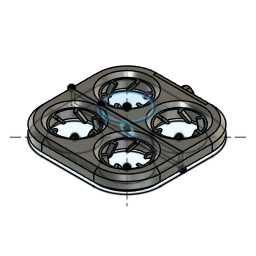
2024_08_05_FlatDrone v2 (Autodesk Fusion 360 design; units mm, degrees)
Autodesk Fusion 360 part; units mm, degrees
sketch "Sketch1" plane through (0, 0, 0) normal (0, 0, 1) x (1, 0, 0)
  line L0 (15.75, 35.75) -> (-15.75, 35.75)
  line L1 (-35.75, 15.75) -> (-35.75, -15.75)
  line L2 (-15.75, -35.75) -> (15.75, -35.75)
  line L3 (35.75, -15.75) -> (35.75, 15.75)
  line L4 (35.75, 35.75) -> (-35.75, -35.75) construction
  line L5 (-35.75, 35.75) -> (35.75, -35.75) construction
  arc A0 (-15.75, 35.75) -> (-35.75, 15.75) centre (-15.75, 15.75) ccw
  arc A1 (35.75, 15.75) -> (15.75, 35.75) centre (15.75, 15.75) ccw
  arc A2 (15.75, -35.75) -> (35.75, -15.75) centre (15.75, -15.75) ccw
  arc A3 (-35.75, -15.75) -> (-15.75, -35.75) centre (-15.75, -15.75) ccw
  line L6 (-27.75, 15.75) -> (-27.75, -15.75) construction
  arc A4 (-27.75, -15.75) -> (-15.75, -27.75) centre (-15.75, -15.75) ccw construction
  line L7 (-15.75, -27.75) -> (15.75, -27.75) construction
  arc A5 (15.75, -27.75) -> (27.75, -15.75) centre (15.75, -15.75) ccw construction
  line L8 (27.75, -15.75) -> (27.75, 15.75) construction
  arc A6 (27.75, 15.75) -> (15.75, 27.75) centre (15.75, 15.75) ccw construction
  line L9 (15.75, 27.75) -> (-15.75, 27.75) construction
  arc A7 (-15.75, 27.75) -> (-27.75, 15.75) centre (-15.75, 15.75) ccw construction
  circle A8 centre (-15.75, 15.75) radius 12
  circle A9 centre (15.75, 15.75) radius 12
  circle A10 centre (15.75, -15.75) radius 12
  circle A11 centre (-15.75, -15.75) radius 12
  dimension "d1" = 71.5
  dimension "d2" = 71.5
  dimension "d3" = 20
  dimension "d4" = -8
  constraint horizontal L0
  constraint perpendicular L0 L1
  constraint parallel L0 L2
  constraint parallel L1 L3
  constraint coincident L4 origin
  constraint coincident L5 origin
  constraint coincident L5.start L1
  constraint coincident L5.start L0
  constraint tangent L1 A0
  constraint tangent L0 A0
  constraint coincident L4.start L0
  constraint coincident L4.start L3
  constraint tangent L0 A1
  constraint tangent L3 A1
  constraint equal A0 A1
  constraint coincident L5.end L3
  constraint coincident L5.end L2
  constraint tangent L3 A2
  constraint tangent L2 A2
  constraint equal A0 A2
  constraint coincident L4.end L2
  constraint coincident L4.end L1
  constraint tangent L2 A3
  constraint tangent L1 A3
  constraint equal A0 A3
  constraint coincident L6.start A8
  constraint coincident L9.end A8
  constraint tangent L9 A8
  constraint coincident L8.end A9
  constraint coincident A6.end A9
  constraint tangent L9 A9
  constraint coincident A5.end A10
  constraint coincident L7.end A10
  constraint tangent L7 A10
  constraint coincident A4.end A11
  constraint coincident L6.end A11
  constraint tangent L6 A11
  measures "d1" distance of L4.end L5.end
  measures "d2" distance of L5.start L4.end
  measures "d3" radius of A0
extrude "Extrude1" add sketch "Sketch1" along normal blind 9 makes body 1
chamfer "Chamfer1" distance 2.3 angle 45 24 edges at (-26.9379, 20.0894, 9) (4.5621, 20.0894, 9) (4.5621, -11.4106, 9) (-26.9379, -11.4106, 9) (35.75, 0, 9) (29.8921, 29.8921, 9) (0, 35.75, 9) (-29.8921, 29.8921, 9) (-35.75, 0, 9) (-29.8921, -29.8921, 9) (0, -35.75, 9) (29.8921, -29.8921, 9) (35.75, 0, 0) (29.8921, 29.8921, 0) (0, 35.75, 0) (-29.8921, 29.8921, 0) (-35.75, 0, 0) (-29.8921, -29.8921, 0) (0, -35.75, 0) (29.8921, -29.8921, 0) (4.5621, 20.0894, 0) (4.5621, -11.4106, 0) (-26.9379, -11.4106, 0) (-26.9379, 20.0894, 0) on bodies 1
sketch "Sketch2" plane through (0, 0, 0) normal (0, 0, 1) x (1, 0, 0)
  circle A0 centre (-15.75, 15.75) radius 12
  point P0 (-15.75, 15.75)
  point P1 (-15.75, 27.75)
  constraint coincident P0 A0.centre
  constraint coincident A0 P1
sketch "Sketch3" plane through (0, 0, 0) normal (1, 0, 0) x (0, 1, 0)
sketch "Sketch4" plane through (0, 0, 0) normal (0, 1, 0) x (1, 0, 0)
  line L0 (-15.75, 0) -> (-12.75, 0)
  line L1 (-12.75, 0) -> (-12.75, -9)
  line L2 (-12.75, -9) -> (-15.75, -9)
  line L3 (-15.75, 0) -> (-18.75, 0)
  line L4 (-18.75, 0) -> (-18.75, -9)
  line L5 (-18.75, -9) -> (-15.75, -9)
  line L6 (-18.75, -9) -> (-12.75, -1.82)
  line L7 (-12.75, 0) -> (-18.75, -7.18)
  point P0 (-15.75, 0)
  dimension "d8" = 3
  dimension "d9" = 9
  dimension "d10" = 3
  constraint horizontal L0
  constraint vertical L1
  constraint horizontal L2
  constraint coincident P0 L0.start
  constraint horizontal L3
  constraint vertical L4
  constraint horizontal L5
  constraint coincident L1 L6.end
  constraint coincident L4 L7.end
  constraint parallel L6 L7
  measures "d8" distance of P0 L0.end
  measures "d9" distance of P0 L2.end
  measures "d10" distance of P0 L3.end
extrude "Extrude2" add sketch "Sketch4" against normal blind 3 separate body contours L1 L4 L6 L7 makes body 2
extrude "Extrude3" add sketch "Sketch4" along normal blind 1 bodies 2
move_body "Move1" bodies 2 to x (1, 0, 0) y (0, 1, 0) z (0, 0, 1) at (0, 27, 0)
pattern_circular "C-Pattern1" count 6 over 360 about axis through (-15.75, 15.75, 0) along (0, 0, 1) of bodies 2 makes body 3 at (-26.8588, 21.009, 3) makes body 4 at (-25.8588, 8.759, 3) makes body 5 at (-14.75, 3.5, 3) makes body 6 at (-5.6412, 8.759, 6) makes body 7 at (-4.6412, 21.009, 6)
extrude "Extrude4" cut sketch "Sketch1" along normal blind 11 bodies 2 3 4 5 6 7
sketch "Sketch5" plane through (0, 0, 0) normal (0, 0, 1) x (1, 0, 0)
  circle A0 centre (-15.75, 15.75) radius 12
  circle A1 centre (-15.75, 15.75) radius 11
  point P0 (-15.75, 15.75)
  dimension "d19" = -1
  constraint coincident P0 A0.centre
extrude "Extrude5" add sketch "Sketch5" along normal blind 9 bodies 2 3 4 5 6 7
mirror "Mirror1" about plane through (0, 0, 0) normal (1, 0, 0) of bodies 2 makes body 8
mirror "Mirror2" about plane through (0, 0, 0) normal (0, 1, 0) of bodies 2 8 makes body 9 at (-3.8096, -14.5552, 3) makes body 10 at (3.8096, -14.5552, 3)
move_body "Move2" bodies 8 2 10 9 to x (0, 1, 0) y (-1, 0, 0) z (0, 0, 1) at (0, 0, 0)
sketch "Sketch6" plane through (0, 0, 0) normal (0, 1, 0) x (1, 0, 0)
  line L0 (-33.45, -9) -> (33.45, -9)
  line L1 (33.45, -9) -> (33.45, 0)
  line L2 (33.45, 0) -> (-33.45, 0)
  line L3 (-33.45, 0) -> (-33.45, -9)
  line L4 (31.45, -2) -> (-31.45, -2)
  line L5 (-31.45, -2) -> (-31.45, -7)
  line L6 (-31.45, -7) -> (31.45, -7)
  line L7 (31.45, -7) -> (31.45, -2)
  point P0 (-33.45, -9)
  point P1 (33.45, 0)
  dimension "d27" = -2
  constraint horizontal L0
  constraint vertical L1
  constraint horizontal L2
  constraint vertical L3
  constraint coincident P1 L1.end
  constraint coincident P0 L0.start
extrude "Extrude6" cut sketch "Sketch6" along normal blind 84 and the other way blind 38 bodies 2 8 9 10
sketch "Sketch7" plane through (0, 0, 0) normal (0, 0, 1) x (1, 0, 0)
  line L0 (-15.75, 35.75) -> (15.75, 35.75)
  line L1 (15.75, 35.75) -> (15.75, 31.7574)
  line L2 (15.75, 31.7574) -> (-15.75, 31.7574)
  line L3 (-15.75, 31.7574) -> (-15.75, 35.75)
  point P0 (-15.75, 35.75)
  constraint horizontal L0
  constraint vertical L1
  constraint horizontal L2
  constraint vertical L3
  constraint coincident P0 L0.start
extrude "Extrude7" cut sketch "Sketch7" along normal blind 16 bodies 1
extrude "Extrude8" add 1 faces at (-15.75, 33.0883, 3.7667) along direction (1, 0, 0) blind 31.5 separate body on bodies 1 makes body 11
combine "Combine1" operation cut target body 1 tool bodies 10 8 9 2 keep tools
sketch "Sketch8" plane through (0, 0, 0) normal (0, 1, 0) x (1, 0, 0)
  line L0 (15.75, 0) -> (-15.75, 0)
  line L1 (-15.75, 0) -> (-15.75, -9)
  line L2 (-15.75, -9) -> (15.75, -9)
  line L3 (15.75, -9) -> (15.75, 0)
  line L4 (15.75, -9) -> (-15.75, 0) construction
  line L5 (-3.7906, -4.5) -> (-3.0667, -6.7281)
  line L6 (-3.0667, -6.7281) -> (-1.1714, -8.1051)
  line L7 (-1.1714, -8.1051) -> (1.1714, -8.1051)
  line L8 (1.1714, -8.1051) -> (3.0667, -6.7281)
  line L9 (3.0667, -6.7281) -> (3.7906, -4.5)
  line L10 (3.7906, -4.5) -> (3.0667, -2.2719)
  line L11 (3.0667, -2.2719) -> (1.1714, -0.8949)
  line L12 (1.1714, -0.8949) -> (-1.1714, -0.8949)
  line L13 (-1.1714, -0.8949) -> (-3.0667, -2.2719)
  line L14 (-3.0667, -2.2719) -> (-3.7906, -4.5)
  line L15 (0.8465, -7.1051) -> (2.216, -6.11)
  line L16 (2.216, -6.11) -> (2.7392, -4.5)
  line L17 (2.7392, -4.5) -> (2.216, -2.89)
  line L18 (2.216, -2.89) -> (0.8465, -1.8949)
  line L19 (0.8465, -1.8949) -> (-0.8465, -1.8949)
  line L20 (-0.8465, -1.8949) -> (-2.216, -2.89)
  line L21 (-2.216, -2.89) -> (-2.7392, -4.5)
  line L22 (-2.7392, -4.5) -> (-2.216, -6.11)
  line L23 (-2.216, -6.11) -> (-0.8465, -7.1051)
  line L24 (-0.8465, -7.1051) -> (0.8465, -7.1051)
  point P0 (15.75, 0)
  point P1 (-15.75, -9)
  point P2 (0, -4.5)
  dimension "d36" = -1
  constraint horizontal L0
  constraint vertical L1
  constraint horizontal L2
  constraint vertical L3
  constraint coincident P1 L1.end
  constraint coincident P0 L0.start
  constraint midpoint L4 P2
extrude "Extrude9" add sketch "Sketch8" along normal blind 3 separate body contours L5 L6 L7 L8 L9 L10 L11 L12 L13 L14 makes body 12
extrude "Extrude10" add sketch "Sketch8" along normal blind 2 contours L15 L16 L17 L18 L19 L20 L21 L22 L23 L24 bodies 12
move_body "Move3" bodies 12 to x (1, 0, 0) y (0, 1, 0) z (0, 0, 1) at (0, 34, 0)
combine "Combine2" operation add target body 11 tool bodies 12
named bodies: "DroneBody", "MotorDownLeft", "MotorTopLeft", "MotorDownRight", "MotorTopRight", "FrontLight"
